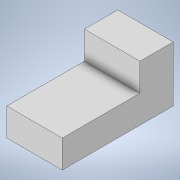
# Autodesk Inventor part: Peça1
Saved by Autodesk Inventor 2021 (Build 250183000, 183)
## iProperties
Created: 2022-02-08
Part Number: Peça1
Material: Genérico
Document SubType Name: Modeling
Designer: aluno
Density: 1 g/cm^3
Appearance: Padrão
Author: aluno
Autodesk Inventor part; units mm, degrees
ref_plane "YZ Plane" through (0, 0, 0) normal (1, 0, 0) x (0, 1, 0)
ref_plane "XZ Plane" through (0, 0, 0) normal (0, 1, 0) x (-1, 0, 0)
ref_plane "XY Plane" through (0, 0, 0) normal (0, 0, 1) x (1, 0, 0)
sketch "Esboço3" plane through (0, 0, 0) normal (0, 0, 1) x (1, 0, 0)
  line L0 (0, 0) -> (60, 0)
  line L1 (60, 0) -> (60, 30)
  line L2 (60, 30) -> (42, 30)
  line L3 (42, 30) -> (42, 15)
  line L4 (42, 15) -> (0, 15)
  line L5 (0, 15) -> (0, 0)
  dimension "d0" = 60
  dimension "d1" = 30
  dimension "d2" = 18
  dimension "d3" = 15
  constraints: 12 end point, 5 perpendicular, 1 horizontal
  measures "d0" distance of L0.start L0.end
  measures "d1" distance of L0.end L1.end
  measures "d2" distance of L1.end L2.end
  measures "d3" distance of L2.end L3.end
extrude "Extrusão1" add sketch "Esboço3" along normal blind 30
